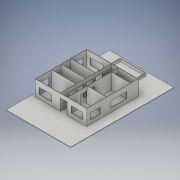
# Autodesk Inventor part: maqueta casa
Saved by Autodesk Inventor 2019 (Build 230136000, 136)
## iProperties
Created: 2022-10-15
Part Number: maqueta casa
Material: Genérico
Document SubType Name: Modeling
Designer: aimar
Density: 1 g/cm^3
Appearance: Valor por defecto
Author: aimar
Autodesk Inventor part; units mm, degrees
ref_plane "YZ Plane" through (0, 0, 0) normal (1, 0, 0) x (0, 1, 0)
sketch "Boceto1" plane through (0, 0, 0) normal (0, 1, 0) x (-1, 0, 0)
  line L0 (-250, 400) -> (250, 400)
  line L1 (250, 400) -> (250, -400)
  line L2 (250, -400) -> (-250, -400)
  line L3 (-250, -400) -> (-250, 400)
  line L4 (-250, 400) -> (250, -400) construction
  line L5 (250, 400) -> (-250, -400) construction
  line L6 (-175, 200) -> (225, 200)
  line L7 (225, 200) -> (225, -200)
  line L8 (225, -200) -> (-175, -200)
  line L9 (-175, -200) -> (-175, 200)
  line L10 (-175, 200) -> (225, -200) construction
  line L11 (225, 200) -> (-175, -200) construction
  point P0 (0, 0)
  point P1 (25, 0)
  dimension "d0" = 500
  dimension "d1" = 800
  dimension "d4" = 400
  dimension "d5" = 400
  dimension "d6" = 200
  dimension "d7" = 75
  constraints: 24 end point, 4 midpoint, 4 parallel, 2 horizontal, 2 perpendicular
  measures "d0" distance of L1.end L2.end
  measures "d1" distance of L0.end L1.end
  measures "d4" distance of L7.end L8.end
  measures "d5" distance of L6.end L7.end
  measures "d6" distance between parallel lines of L2 L8
  measures "d7" distance between parallel lines of L3 L9
extrude "Extrusión1" add sketch "Boceto1" along normal blind 4 contours L0 L1 L2 L3 | L6 L7 L8 L9
sketch "Boceto2" plane through (0, 4, 0) normal (0, 1, 0) x (1, 0, 0)
  line L0 (175, -200) -> (-225, -200)
  line L1 (-225, -200) -> (-225, 200)
  line L2 (-225, 200) -> (175, 200)
  line L3 (175, 200) -> (175, -200)
  line L4 (175, -200) -> (-225, 200) construction
  line L5 (-225, -200) -> (175, 200) construction
  line L6 (250, -400) -> (250, 400) projected
  line L7 (250, 400) -> (-250, 400) projected
  line L8 (-221, -196) -> (-34, -196)
  line L9 (-34, -196) -> (-34, -76)
  line L10 (-34, -76) -> (-221, -76)
  line L11 (-221, -76) -> (-221, -196)
  line L12 (171, -196) -> (26, -196)
  line L13 (26, -196) -> (26, -46)
  line L14 (26, -46) -> (171, -46)
  line L15 (171, -46) -> (171, -196)
  line L16 (171, 196) -> (26, 196)
  line L17 (26, 196) -> (26, -42)
  line L18 (26, -42) -> (171, -42)
  line L19 (171, -42) -> (171, 196)
  line L20 (-34, -72) -> (-221, -72)
  line L21 (-221, -72) -> (-221, 72)
  line L22 (-221, 72) -> (-34, 72)
  line L23 (-34, 72) -> (-34, -72)
  line L24 (-34, 76) -> (-221, 76)
  line L25 (-221, 76) -> (-221, 196)
  line L26 (-221, 196) -> (-34, 196)
  line L27 (-34, 196) -> (-34, 76)
  line L28 (-30, 196) -> (22, 196)
  line L29 (22, 196) -> (22, 122)
  line L30 (-30, 122) -> (-30, 196)
  line L31 (-34, 0) -> (-34, -2)
  line L32 (-34, -2) -> (-34, 2)
  line L33 (-34, 2) -> (-221, 2)
  line L34 (-221, -2) -> (-34, -2)
  line L35 (-30, -200) -> (-30, 122)
  line L36 (22, 122) -> (22, -200)
  line L37 (-30, -196) -> (22, -196)
  line L38 (26, 196) -> (26, 144)
  line L39 (26, 144) -> (26, 140)
  line L40 (26, 140) -> (171, 140)
  line L41 (171, 144) -> (26, 144)
  point P0 (0, 0)
  point P1 (-25, 0)
  point P2 (-30, 126)
  point P3 (22, 126)
  dimension "d8" = 400
  dimension "d9" = 400
  dimension "d10" = 75
  dimension "d11" = 200
  dimension "d12" = 4
  dimension "d13" = 4
  dimension "d14" = 4
  dimension "d15" = 4
  dimension "d16" = 4
  dimension "d17" = 60
  dimension "d18" = 145
  dimension "d19" = 150
  dimension "d20" = 120
  dimension "d21" = 120
  dimension "d22" = 4
  dimension "d23" = 4
  dimension "d24" = 2
  dimension "d25" = 4
  dimension "d27" = 4
  dimension "d39" = 52
  dimension "d40" = 4
  constraints: 80 end point, 24 point on line, 15 parallel, 11 perpendicular, 7 horizontal, 3 midpoint, 1 collinear
  measures "d8" distance of L1.end L2.end
  measures "d9" distance of L0.end L1.end
  measures "d10" distance between parallel lines of L6 L3
  measures "d11" distance between parallel lines of L7 L2
  measures "d12" distance between parallel lines of L0 L12
  measures "d13" distance between parallel lines of L2 L16
  measures "d14" distance between parallel lines of L18 L14
  measures "d15" distance between parallel lines of L20 L10
  measures "d16" distance between parallel lines of L24 L22
  measures "d17" distance between parallel lines of L27 L17
  measures "d18" distance of L12.start L12.end
  measures "d19" distance of L12.end L13.end
  measures "d20" distance of L26.end L24.start
  measures "d21" distance of L8.end L9.end
  measures "d22" distance between parallel lines of L27 L30
  measures "d23" distance between parallel lines of L17 L29
  measures "d24" distance of L31.start L31.end
  measures "d25" distance of L31.end L32.end
  measures "d27" distance between parallel lines of L2 L28
  measures "d39" distance of L16.end L38.end
  measures "d40" distance of L38.end L39.end
ref_plane "Plano de trabajo1" through (-225, 4, 200) normal (0, 0, 1) x (1, 0, 0)
sketch "Boceto3" plane through (-225, 4, 200) normal (0, 0, 1) x (1, 0, 0)
  line L0 (195, 0) -> (195, 120) projected
  line L1 (247, 0) -> (247, 120) projected
  line L2 (195, 0) -> (247, 0)
  line L3 (247, 0) -> (247, 90)
  line L4 (247, 90) -> (195, 90)
  line L5 (195, 90) -> (195, 0)
  point P0 (225, -4)
  dimension "d31" = 90
  constraints: 8 end point, 2 parallel, 1 horizontal, 1 perpendicular, 1 point on line
  measures "d31" distance of L3.end L2.end
extrude "Extrusión3" cut sketch "Boceto3" against normal blind 120
ref_plane "Plano de trabajo2" through (-30, 4, 200) normal (1, 0, 0) x (0, 0, -1)
sketch "Boceto4" plane through (-30, 4, 200) normal (1, 0, 0) x (0, 0, -1)
  line L0 (124, 0) -> (124, 120) projected
  line L1 (124, 0) -> (72, 0)
  line L2 (72, 0) -> (72, 90)
  line L3 (72, 90) -> (124, 90)
  line L4 (124, 90) -> (124, 0)
  line L5 (0, 0) -> (400, 0) projected
  line L6 (129.886, 90) -> (181.886, 90)
  line L7 (181.886, 90) -> (181.886, 0)
  line L8 (181.886, 0) -> (129.886, 0)
  line L9 (129.886, 0) -> (129.886, 90)
  line L10 (202, 0) -> (202, 120) projected
  line L11 (202, 0) -> (254, 0)
  line L12 (254, 0) -> (254, 90)
  line L13 (254, 90) -> (202, 90)
  line L14 (202, 90) -> (202, 0)
  line L15 (276, 0) -> (276, 120) projected
  line L16 (396, 0) -> (276, 0) projected
  line L17 (276, 90) -> (328, 90)
  line L18 (328, 90) -> (328, 0)
  line L19 (328, 0) -> (276, 0)
  line L20 (276, 0) -> (276, 90)
  point P0 (200, -4)
  dimension "d34" = 52
  dimension "d35" = 90
  dimension "d36" = 52
  dimension "d37" = 52
  dimension "d38" = 52
  constraints: 32 end point, 8 parallel, 6 point on line, 4 horizontal, 4 perpendicular
  measures "d34" distance of L2.end L3.end
  measures "d35" distance of L1.end L2.end
  measures "d36" distance of L7.end L8.end
  measures "d37" distance of L13.end L12.end
  measures "d38" distance of L18.end L19.end
extrude "Extrusión4" add sketch "Boceto2" along normal blind 120 contours L0 L36 L29 L28 L30 L35 L1 L2 L3 | L0 L35 L37 L36 | L19 L40 L17 L41 | L34 L21 L33 L23
extrude "Extrusión5" cut sketch "Boceto4" against normal blind 120
sketch "Boceto5" plane through (22, 4, -196) normal (-1, 0, 0) x (0, 0, 1)
  line L0 (596, 0) -> (-204, 0) projected
  line L1 (0, 0) -> (52, 0)
  line L2 (52, 0) -> (52, 90)
  line L3 (52, 90) -> (0, 90)
  line L4 (0, 90) -> (0, 0)
  line L5 (238, 0) -> (238, 120) projected
  line L6 (238, 90) -> (186, 90)
  line L7 (186, 90) -> (186, 0)
  line L8 (186, 0) -> (238, 0)
  line L9 (238, 0) -> (238, 90)
  line L10 (242, 0) -> (242, 120) projected
  line L11 (242, 0) -> (392, 0) projected
  line L12 (242, 90) -> (294, 90)
  line L13 (294, 90) -> (294, 0)
  line L14 (294, 0) -> (242, 0)
  line L15 (242, 0) -> (242, 90)
  line L16 (0, 0) -> (0, 120) projected
  point P0 (196, -4)
  dimension "d45" = 52
  dimension "d46" = 90
  dimension "d47" = 52
  dimension "d48" = 52
  dimension "d108" = 0
  constraints: 24 end point, 7 point on line, 6 parallel, 3 horizontal, 3 perpendicular
  measures "d45" distance of L3.end L2.end
  measures "d46" distance of L2.end L1.end
  measures "d47" distance of L8.end L7.end
  measures "d48" distance of L13.end L14.end
  measures "d108" distance between parallel lines of L16 L4
extrude "Extrusión6" cut sketch "Boceto5" against normal blind 120
sketch "Boceto6" plane through (-225, 4, 200) normal (0, 0, 1) x (1, 0, 0)
  line L0 (195, 0) -> (247, 0) projected
  line L1 (247, 0) -> (247, 120) projected
  line L2 (195, 0) -> (247, 0)
  line L3 (247, 0) -> (247, 90)
  line L4 (247, 90) -> (195, 90)
  line L5 (195, 90) -> (195, 0)
  point P0 (225, -4)
  dimension "d51" = 90
  constraints: 8 end point, 2 parallel, 1 horizontal, 1 perpendicular, 1 point on line
  measures "d51" distance of L3.end L2.end
extrude "Extrusión7" cut sketch "Boceto6" against normal blind 120
sketch "Boceto7" plane through (0, 4, 0) normal (0, 1, 0) x (1, 0, 0)
  line L0 (-135, 240) -> (65, 240)
  line L1 (65, 240) -> (65, 370)
  line L2 (65, 370) -> (-135, 370)
  line L3 (-135, 370) -> (-135, 240)
  line L4 (175, 200) -> (-225, 200) projected
  line L5 (-250, 400) -> (-250, -400) projected
  line L6 (61, 244) -> (-131, 244)
  line L7 (-131, 244) -> (-131, 366)
  line L8 (-131, 366) -> (61, 366)
  line L9 (61, 366) -> (61, 244)
  line L10 (61, 244) -> (-131, 366) construction
  line L11 (-131, 244) -> (61, 366) construction
  point P0 (0, 0)
  point P1 (-35, 305)
  dimension "d54" = 200
  dimension "d55" = 130
  dimension "d56" = 40
  dimension "d57" = 115
  dimension "d58" = 192
  dimension "d59" = 122
  dimension "d60" = 4
  dimension "d61" = 4
  constraints: 20 end point, 4 parallel, 2 horizontal, 2 midpoint, 2 perpendicular
  measures "d54" distance of L2.end L1.end
  measures "d55" distance of L1.end L0.end
  measures "d56" distance between parallel lines of L4 L0
  measures "d57" distance between parallel lines of L5 L3
  measures "d58" distance of L7.end L8.end
  measures "d59" distance of L6.end L7.end
  measures "d60" distance between parallel lines of L2 L8
  measures "d61" distance between parallel lines of L1 L9
extrude "Extrusión8" add sketch "Boceto7" along normal blind 20
sketch "Boceto8" plane through (-225, 4, 200) normal (0, 0, 1) x (1, 0, 0)
  line L0 (30, 30) -> (130, 30)
  line L1 (130, 30) -> (130, 80)
  line L2 (130, 80) -> (30, 80)
  line L3 (30, 80) -> (30, 30)
  line L4 (30, 30) -> (130, 80) construction
  line L5 (130, 30) -> (30, 80) construction
  line L6 (195, 0) -> (0, 0) projected
  line L7 (0, 0) -> (0, 120) projected
  point P0 (225, -4)
  point P1 (80, 55)
  dimension "d64" = 100
  dimension "d65" = 50
  dimension "d66" = 30
  dimension "d67" = 30
  constraints: 12 end point, 2 midpoint, 2 parallel, 1 horizontal, 1 perpendicular
  measures "d64" distance of L2.end L1.end
  measures "d65" distance of L1.end L0.end
  measures "d66" distance between parallel lines of L6 L0
  measures "d67" distance between parallel lines of L7 L3
extrude "Extrusión9" cut sketch "Boceto8" against normal blind 10
sketch "Boceto9" plane through (-225, 4, -200) normal (-1, 0, 0) x (0, 0, 1)
  line L0 (295, 30) -> (370, 30)
  line L1 (370, 30) -> (370, 80)
  line L2 (370, 80) -> (295, 80)
  line L3 (295, 80) -> (295, 30)
  line L4 (295, 30) -> (370, 80) construction
  line L5 (370, 30) -> (295, 80) construction
  line L6 (400, 0) -> (400, 120) projected
  line L7 (400, 0) -> (0, 0) projected
  point P0 (200, -4)
  point P1 (332.5, 55)
  dimension "d70" = 75
  dimension "d71" = 50
  dimension "d72" = 30
  dimension "d73" = 30
  constraints: 12 end point, 2 midpoint, 2 parallel, 1 horizontal, 1 perpendicular
  measures "d70" distance of L2.end L1.end
  measures "d71" distance of L1.end L0.end
  measures "d72" distance between parallel lines of L1 L6
  measures "d73" distance between parallel lines of L7 L0
extrude "Extrusión10" cut sketch "Boceto9" against normal blind 10
sketch "Boceto10" plane through (-225, 4, -200) normal (-1, 0, 0) x (0, 0, 1)
  line L0 (30, 30) -> (105, 30)
  line L1 (105, 30) -> (105, 80)
  line L2 (105, 80) -> (30, 80)
  line L3 (30, 80) -> (30, 30)
  line L4 (30, 30) -> (105, 80) construction
  line L5 (105, 30) -> (30, 80) construction
  line L6 (0, 0) -> (0, 120) projected
  line L7 (-200, 0) -> (600, 0) projected
  line L8 (219.5, 30) -> (254.5, 30)
  line L9 (254.5, 30) -> (254.5, 80)
  line L10 (254.5, 80) -> (219.5, 80)
  line L11 (219.5, 80) -> (219.5, 30)
  line L12 (219.5, 30) -> (254.5, 80) construction
  line L13 (254.5, 30) -> (219.5, 80) construction
  line L14 (272, 0) -> (272, 120) projected
  point P0 (200, -4)
  point P1 (67.5, 55)
  point P2 (237, 55)
  dimension "d76" = 75
  dimension "d77" = 50
  dimension "d78" = 30
  dimension "d79" = 30
  dimension "d80" = 35
  dimension "d81" = 50
  dimension "d82" = 30
  dimension "d83" = 17.5
  constraints: 24 end point, 4 midpoint, 4 parallel, 2 horizontal, 2 perpendicular
  measures "d76" distance of L2.end L1.end
  measures "d77" distance of L1.end L0.end
  measures "d78" distance between parallel lines of L6 L3
  measures "d79" distance between parallel lines of L7 L0
  measures "d80" distance of L10.end L9.end
  measures "d81" distance of L9.end L8.end
  measures "d82" distance between parallel lines of L7 L8
  measures "d83" distance between parallel lines of L14 L9
extrude "Extrusión11" cut sketch "Boceto10" against normal blind 10
sketch "Boceto11" plane through (-225, 4, 200) normal (0, 0, 1) x (1, 0, 0)
  line L0 (280, 30) -> (370, 30)
  line L1 (370, 30) -> (370, 80)
  line L2 (370, 80) -> (280, 80)
  line L3 (280, 80) -> (280, 30)
  line L4 (280, 30) -> (370, 80) construction
  line L5 (370, 30) -> (280, 80) construction
  line L6 (-25, 0) -> (475, 0) projected
  line L7 (400, 0) -> (400, 120) projected
  point P0 (225, -4)
  point P1 (325, 55)
  dimension "d86" = 90
  dimension "d88" = 30
  dimension "d89" = 50
  dimension "d90" = 30
  constraints: 12 end point, 2 midpoint, 2 parallel, 1 horizontal, 1 perpendicular
  measures "d86" distance of L0.start L0.end
  measures "d88" distance between parallel lines of L6 L0
  measures "d89" distance between parallel lines of L2 L0
  measures "d90" distance between parallel lines of L7 L1
extrude "Extrusión12" cut sketch "Boceto11" against normal blind 10
sketch "Boceto12" plane through (175, 4, -200) normal (0, 0, -1) x (-1, 0, 0)
  line L0 (270, 30) -> (370, 30)
  line L1 (370, 30) -> (370, 80)
  line L2 (370, 80) -> (270, 80)
  line L3 (270, 80) -> (270, 30)
  line L4 (270, 30) -> (370, 80) construction
  line L5 (370, 30) -> (270, 80) construction
  line L6 (400, 0) -> (400, 120) projected
  line L7 (-75, 0) -> (425, 0) projected
  point P0 (175, -4)
  point P1 (320, 55)
  dimension "d93" = 100
  dimension "d94" = 50
  dimension "d95" = 30
  dimension "d96" = 30
  constraints: 12 end point, 2 midpoint, 2 parallel, 1 horizontal, 1 perpendicular
  measures "d93" distance of L2.end L1.end
  measures "d94" distance of L1.end L0.end
  measures "d95" distance between parallel lines of L6 L1
  measures "d96" distance between parallel lines of L7 L0
extrude "Extrusión13" cut sketch "Boceto12" against normal blind 10
sketch "Boceto13" plane through (175, 4, 200) normal (1, 0, 0) x (0, 0, -1)
  line L0 (30, 30) -> (105, 30) projected
  line L1 (105, 80) -> (30, 80) projected
  line L2 (30, 30) -> (105, 30)
  line L3 (105, 30) -> (105, 80)
  line L4 (105, 80) -> (30, 80)
  line L5 (30, 80) -> (30, 30)
  point P0 (200, -4)
  constraints: 8 end point, 2 parallel, 1 horizontal, 1 perpendicular
extrude "Extrusión14" cut sketch "Boceto13" against normal blind 10
sketch "Boceto14" plane through (175, 4, 200) normal (1, 0, 0) x (0, 0, -1)
  line L0 (186.5, 30) -> (311.5, 30)
  line L1 (311.5, 30) -> (311.5, 80)
  line L2 (311.5, 80) -> (186.5, 80)
  line L3 (186.5, 80) -> (186.5, 30)
  line L4 (186.5, 30) -> (311.5, 80) construction
  line L5 (311.5, 30) -> (186.5, 80) construction
  line L6 (-200, 0) -> (600, 0) projected
  line L7 (158, 0) -> (158, 120) projected
  point P0 (200, -4)
  point P1 (249, 55)
  dimension "d101" = 125
  dimension "d102" = 50
  dimension "d103" = 30
  dimension "d105" = 91
  constraints: 12 end point, 2 midpoint, 2 parallel, 1 horizontal, 1 perpendicular
  measures "d101" distance of L2.end L1.end
  measures "d102" distance of L1.end L0.end
  measures "d103" distance between parallel lines of L6 L0
  measures "d105" distance from line of L7 point (249, 55)
extrude "Extrusión15" cut sketch "Boceto14" against normal blind 10
